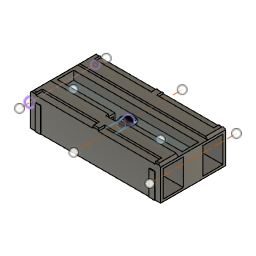
Pièce garage v32 (Autodesk Fusion 360 design; units mm, degrees)
Autodesk Fusion 360 part; units mm, degrees
sketch "Esquisse3" plane through (0, 0, 0) normal (0, 0, 1) x (1, 0, 0)
  line L0 (60, -30) -> (-60, -30)
  line L1 (-60, -30) -> (-60, 30)
  line L2 (-60, 30) -> (60, 30)
  line L3 (60, 30) -> (60, -30)
  line L4 (60, -30) -> (-60, 30) construction
  line L5 (-60, -30) -> (60, 30) construction
  dimension "d3" = 120
  dimension "d4" = 60
  constraint horizontal L0
  constraint perpendicular L0 L1
  constraint parallel L0 L2
  constraint parallel L1 L3
  constraint coincident L4 origin
  constraint coincident L5 origin
  measures "d3" distance of L1.end L2.end
  measures "d4" distance of L0.end L1.end
extrude "Extrusion1" add sketch "Esquisse3" along normal blind 30.7
sketch "Esquisse4" plane through (0, 0, 30.7) normal (0, 0, 1) x (-1, 0, 0)
  line L0 (-60, -30) -> (60, -30)
  line L1 (60, -30) -> (60, 30)
  line L2 (60, 30) -> (-60, 30)
  line L3 (-60, 30) -> (-60, -30)
  line L4 (57.5, 7.5) -> (-57.5, 7.5)
  line L5 (-57.5, 7.5) -> (-57.5, -7.5)
  line L6 (-57.5, -7.5) -> (57.5, -7.5)
  line L7 (57.5, -7.5) -> (57.5, 7.5)
  line L8 (57.5, 7.5) -> (-57.5, -7.5) construction
  line L9 (-57.5, 7.5) -> (57.5, -7.5) construction
  dimension "d7" = 115
  dimension "d8" = 15
  constraint horizontal L4
  constraint perpendicular L4 L5
  constraint parallel L4 L6
  constraint parallel L5 L7
  constraint coincident L8 origin
  constraint coincident L9 origin
  measures "d7" distance of L5.end L6.end
  measures "d8" distance of L4.end L5.end
extrude "Extrusion2" cut sketch "Esquisse4" against normal blind 10 contours L4 L5 L6 L7
sketch "Esquisse5" plane through (0, 0, 20.7) normal (0, 0, 1) x (-1, 0, 0)
  line L0 (57.5, -7.5) -> (57.5, 7.5)
  line L1 (57.5, 7.5) -> (-57.5, 7.5)
  line L2 (-57.5, 7.5) -> (-57.5, -7.5)
  line L3 (-57.5, -7.5) -> (57.5, -7.5)
  circle A0 centre (0, 0) radius 6.15
  circle A1 centre (50.4, 0) radius 3.1
  spline S0 degree 5 poles (60, -40) (60, -36.8) (60, -30.4) (60, -20.8) (60, -8) (60, 8) (60, 20.8) (60, 30.4) (60, 36.8) (60, 40) knots 0 0 0 0 0 0 0.2 0.4 0.6 0.8 1 1 1 1 1 1 construction
  line L4 (60, 30) -> (60, -30) construction
  circle A2 centre (-30, 0) radius 3.1
  spline S1 degree 5 poles (-60, -40) (-60, -36.8) (-60, -30.4) (-60, -20.8) (-60, -8) (-60, 8) (-60, 20.8) (-60, 30.4) (-60, 36.8) (-60, 40) knots 0 0 0 0 0 0 0.2 0.4 0.6 0.8 1 1 1 1 1 1 construction
  line L5 (-60, 31.84) -> (-60, 48.16)
  line L6 (0, -50) -> (0, 50) construction
  line L7 (-4.45, 16) -> (4.45, 16)
  line L8 (4.45, 16) -> (4.45, -3.7)
  line L9 (4.45, -3.7) -> (-4.45, -3.7)
  line L10 (-4.45, -3.7) -> (-4.45, 16)
  line L11 (-4.45, 16) -> (4.45, -3.7) construction
  line L12 (4.45, 16) -> (-4.45, -3.7) construction
  point P0 (0, 6.15)
  dimension "d11" = 12.3
  dimension "d12" = 6.2
  dimension "d13" = 9.6
  dimension "d14" = 6.2
  dimension "d15" = 30
  dimension "d16" = 8.9
  dimension "d17" = 16
  constraint coincident A0.centre origin
  constraint midpoint S1.end L5
  constraint vertical L6
  constraint horizontal L7
  constraint perpendicular L7 L8
  constraint parallel L7 L9
  constraint parallel L8 L10
  constraint coincident L11 P0
  constraint coincident L12 P0
  constraint coincident A0 P0
  constraint coincident L6 P0
  measures "d11" diameter of A0
  measures "d12" diameter of A1
  measures "d13" distance of A1.centre L4
  measures "d14" diameter of A2
  measures "d15" distance of A2.centre L5
  measures "d16" distance of L8.end L9.end
  measures "d17" distance of L7 A0.centre
extrude "Extrusion3" cut sketch "Esquisse5" against normal blind 30.574 contours A1
extrude "Extrusion4" cut sketch "Esquisse5" against normal blind 30.574 contours A0 L8 L9 L10 picked at (-0.0399, -4.5163)
extrude "Extrusion5" cut sketch "Esquisse5" against normal blind 30.574 contours A0 L8 L9 L10 picked at (-0.1506, -0.4222)
extrude "Extrusion6" cut sketch "Esquisse5" against normal blind 30.574 contours L1 A0 L8 L10
extrude "Extrusion7" cut sketch "Esquisse5" against normal blind 30.574 contours L1 L7 L8 L10
extrude "Extrusion8" cut sketch "Esquisse5" along normal blind 22.36 contours L1 L7 L8 L10
extrude "Extrusion9" cut sketch "Esquisse5" against normal blind 30.574 contours A2
sketch "Esquisse6" plane through (0, 0, 30.7) normal (0, 0, 1) x (-1, 0, 0)
  line L0 (-60, -30) -> (60, -30)
  line L1 (60, -30) -> (60, 30)
  line L2 (60, 30) -> (-60, 30)
  line L3 (-60, 30) -> (-60, -30)
  line L4 (-4.45, 7.5) -> (-4.45, 16)
  line L5 (-4.45, 16) -> (4.45, 16)
  line L6 (4.45, 16) -> (4.45, 7.5)
  line L7 (4.45, 7.5) -> (57.5, 7.5)
  line L8 (57.5, 7.5) -> (57.5, -7.5)
  line L9 (57.5, -7.5) -> (-57.5, -7.5)
  line L10 (-57.5, -7.5) -> (-57.5, 7.5)
  line L11 (-57.5, 7.5) -> (-4.45, 7.5)
  line L12 (-60, -13.5) -> (60, -13.5)
  line L13 (60, -13.5) -> (60, 13.5)
  line L14 (60, 13.5) -> (-60, 13.5)
  line L15 (-60, 13.5) -> (-60, -13.5)
  line L16 (-60, -13.5) -> (60, 13.5) construction
  line L17 (60, -13.5) -> (-60, 13.5) construction
  line L18 (0, -50) -> (0, 50) construction
  line L19 (2.5, -50) -> (2.5, 50) construction
  line L20 (-2.5, -50) -> (-2.5, 50) construction
  line L21 (60, -50) -> (60, 50) construction
  line L22 (-60, -50) -> (-60, 50) construction
  line L23 (-60, -50) -> (-60, 50) construction
  line L24 (-55, -50) -> (-55, 50) construction
  line L25 (60, -50) -> (60, 50) construction
  line L26 (55, -50) -> (55, 50) construction
  line L27 (55, -30) -> (2.5, -30)
  line L28 (2.5, -30) -> (2.5, -24)
  line L29 (2.5, -24) -> (55, -24)
  line L30 (55, -24) -> (55, -30)
  line L31 (-2.5, -30) -> (-55, -30)
  line L32 (-55, -30) -> (-55, -24)
  line L33 (-55, -24) -> (-2.5, -24)
  line L34 (-2.5, -24) -> (-2.5, -30)
  line L35 (55, 30) -> (2.5, 30)
  line L36 (2.5, 30) -> (2.5, 24)
  line L37 (2.5, 24) -> (55, 24)
  line L38 (55, 24) -> (55, 30)
  line L39 (-2.5, 30) -> (-55, 30)
  line L40 (-55, 30) -> (-55, 24)
  line L41 (-55, 24) -> (-2.5, 24)
  line L42 (-2.5, 24) -> (-2.5, 30)
  dimension "d32" = 120
  dimension "d33" = 27
  dimension "d34" = 6
  dimension "d35" = 6
  dimension "d36" = 6
  dimension "d37" = 6
  constraint horizontal L12
  constraint perpendicular L12 L13
  constraint parallel L12 L14
  constraint parallel L13 L15
  constraint coincident L16 origin
  constraint coincident L17 origin
  constraint perpendicular L14 L18
  constraint perpendicular L2 L21
  constraint horizontal L27
  constraint vertical L28
  constraint horizontal L29
  constraint vertical L30
  constraint coincident L26 L27.start
  constraint coincident L0 L27.start
  constraint horizontal L31
  constraint vertical L32
  constraint horizontal L33
  constraint vertical L34
  constraint coincident L20 L31.start
  constraint coincident L0 L31.start
  constraint horizontal L35
  constraint vertical L36
  constraint horizontal L37
  constraint vertical L38
  constraint coincident L26 L35.start
  constraint coincident L2 L35.start
  constraint horizontal L39
  constraint vertical L40
  constraint horizontal L41
  constraint vertical L42
  constraint coincident L20 L39.start
  constraint coincident L2 L39.start
  measures "d32" distance of L13.end L14.end
  measures "d33" distance of L12.end L13.end
  measures "d34" distance of L27.start L29.end
  measures "d35" distance of L31.start L33.end
  measures "d36" distance of L35.start L37.end
  measures "d37" distance of L39.start L41.end
extrude "Extrusion10" cut sketch "Esquisse6" against normal blind 2 contours L0 L27 L28 L29 L30
extrude "Extrusion12" cut sketch "Esquisse6" against normal blind 2 contours L0 L31 L32 L33 L34
extrude "Extrusion13" cut sketch "Esquisse6" against normal blind 2 contours L2 L39 L40 L41 L42
extrude "Extrusion14" cut sketch "Esquisse6" against normal blind 2 contours L2 L35 L36 L37 L38
extrude "Extrusion15" cut sketch "Esquisse6" against normal blind 2 contours L1 L3 L4 L6 L7 L8 L9 L10 L11 L12 L13 L14 L15
sketch "Esquisse8" plane through (60, 0, 0) normal (1, 0, 0) x (0, 1, 0)
  line L0 (-13.5, 28.7) -> (-13.5, 30.7)
  line L1 (-13.5, 30.7) -> (-30, 30.7)
  line L2 (-30, 30.7) -> (-30, 0)
  line L3 (-30, 0) -> (30, 0)
  line L4 (30, 0) -> (30, 30.7)
  line L5 (30, 30.7) -> (13.5, 30.7)
  line L6 (13.5, 30.7) -> (13.5, 28.7)
  line L7 (13.5, 28.7) -> (-13.5, 28.7)
  line L8 (-40, 26.5) -> (40, 26.5) construction
  line L9 (-40.0872, 2.1) -> (40, 2.1) construction
  line L10 (27.5, 40.0232) -> (27.5, -9.9768) construction
  line L11 (-27.5, -10) -> (-27.5, 40) construction
  line L12 (9, 40.0232) -> (9, -10) construction
  line L13 (-9, 40) -> (-9, -10) construction
  line L14 (-27.5, 26.5) -> (-9, 26.5)
  line L15 (-9, 26.5) -> (-9, 2.1)
  line L16 (-9, 2.1) -> (-27.5, 2.1)
  line L17 (-27.5, 2.1) -> (-27.5, 26.5)
  line L18 (9, 2.1) -> (27.5, 2.1)
  line L19 (27.5, 2.1) -> (27.5, 26.5)
  line L20 (27.5, 26.5) -> (9, 26.5)
  line L21 (9, 26.5) -> (9, 2.1)
  dimension "d50" = 4.2
  dimension "d51" = 2.1
  dimension "d52" = 2.5
  dimension "d53" = 2.5
  dimension "d54" = 18.5
  dimension "d55" = 18.5
  constraint horizontal L8
  constraint perpendicular L4 L9
  constraint perpendicular L3 L10
  constraint perpendicular L1 L11
  constraint parallel L10 L12
  constraint vertical L13
  constraint horizontal L14
  constraint vertical L15
  constraint horizontal L16
  constraint vertical L17
  constraint coincident L13 L15.end
  constraint coincident L9 L15.end
  constraint coincident L11 L14.start
  constraint coincident L8 L14.start
  constraint horizontal L18
  constraint vertical L19
  constraint horizontal L20
  constraint vertical L21
  constraint coincident L8 L19.end
  constraint coincident L10 L19.end
  constraint coincident L9 L18.start
  constraint coincident L12 L18.start
  measures "d50" distance of L1 L8
  measures "d51" distance of L3 L9
  measures "d52" distance of L4 L10
  measures "d53" distance of L2 L11
  measures "d54" distance of L10.start L12.start
  measures "d55" distance of L11 L13
extrude "Extrusion16" cut sketch "Esquisse8" against normal blind 120 contours L14 L15 L16 L17
extrude "Extrusion17" cut sketch "Esquisse8" against normal blind 120 contours L18 L19 L20 L21
sketch "Esquisse9" plane through (0, -30, 0) normal (0, -1, 0) x (1, 0, 0)
  line L0 (-55, 28.7) -> (-55, 30.7)
  line L1 (-55, 30.7) -> (-60, 30.7)
  line L2 (-60, 30.7) -> (-60, 0)
  line L3 (-60, 0) -> (60, 0)
  line L4 (60, 0) -> (60, 30.7)
  line L5 (60, 30.7) -> (55, 30.7)
  line L6 (55, 30.7) -> (55, 28.7)
  line L7 (55, 28.7) -> (2.5, 28.7)
  line L8 (2.5, 28.7) -> (2.5, 30.7)
  line L9 (2.5, 30.7) -> (-2.5, 30.7)
  line L10 (-2.5, 30.7) -> (-2.5, 28.7)
  line L11 (-2.5, 28.7) -> (-55, 28.7)
  line L12 (-55, 50) -> (-55, -20) construction
  line L13 (-50.2, 50) -> (-50.2, -20) construction
  line L14 (-75, 0) -> (75, 0) construction
  line L15 (-75, 23) -> (75, 23) construction
  line L16 (-50.2, 50) -> (-50.2, -20) construction
  line L17 (-55, 50) -> (-55, -20) construction
  line L18 (55, 50) -> (55, -20) construction
  line L19 (49.8, 50) -> (49.8, -20) construction
  line L20 (-55, 23) -> (-50.2, 23)
  line L21 (-50.2, 23) -> (-50.2, 0)
  line L22 (-50.2, 0) -> (-55, 0)
  line L23 (-55, 0) -> (-55, 23)
  line L24 (55, 0) -> (49.8, 0)
  line L25 (49.8, 0) -> (49.8, 23)
  line L26 (49.8, 23) -> (55, 23)
  line L27 (55, 23) -> (55, 0)
  dimension "d60" = 4.8
  dimension "d61" = 23
  dimension "d62" = 4.8
  constraint perpendicular L11 L12
  constraint perpendicular L11 L13
  constraint parallel L3 L14
  constraint perpendicular L4 L15
  constraint horizontal L20
  constraint vertical L21
  constraint horizontal L22
  constraint vertical L23
  constraint coincident L14 L21.end
  constraint coincident L13 L21.end
  constraint coincident L3 L21.end
  constraint coincident L15 L20.start
  constraint coincident L12 L20.start
  constraint horizontal L24
  constraint vertical L25
  constraint horizontal L26
  constraint vertical L27
  constraint coincident L15 L25.end
  constraint coincident L19 L25.end
  constraint coincident L14 L24.start
  constraint coincident L18 L24.start
  measures "d60" distance of L12 L13
  measures "d61" distance of L14 L15
  measures "d62" distance of L16 L17
extrude "Extrusion18" add sketch "Esquisse9" along normal blind 0.5 contours L3 L24 L25 L26 L27
extrude "Extrusion19" add sketch "Esquisse9" along normal blind 0.5 contours L3 L20 L21 L22 L23
sketch "Esquisse10" plane through (0, 30, 0) normal (0, 1, 0) x (-1, 0, 0)
  line L0 (-2.5, 30.7) -> (-2.5, 28.7)
  line L1 (-2.5, 28.7) -> (-55, 28.7)
  line L2 (-55, 28.7) -> (-55, 30.7)
  line L3 (-55, 30.7) -> (-60, 30.7)
  line L4 (-60, 30.7) -> (-60, 0)
  line L5 (-60, 0) -> (60, 0)
  line L6 (60, 0) -> (60, 30.7)
  line L7 (60, 30.7) -> (55, 30.7)
  line L8 (55, 30.7) -> (55, 28.7)
  line L9 (55, 28.7) -> (2.5, 28.7)
  line L10 (2.5, 28.7) -> (2.5, 30.7)
  line L11 (2.5, 30.7) -> (-2.5, 30.7)
  line L12 (-75, 0) -> (75, 0) construction
  line L13 (-55, 35) -> (-55, -5)
  line L14 (-50, 50) -> (-50, -20) construction
  line L15 (-55, 50) -> (-55, -20) construction
  line L16 (55, 50) -> (55, -20) construction
  line L17 (50, 50) -> (50, -20) construction
  line L18 (-74.8741, 23.108) -> (75, 23.108) construction
  line L19 (-55, 23.108) -> (-50, 23.108)
  line L20 (-50, 23.108) -> (-50, 0)
  line L21 (-50, 0) -> (-55, 0)
  line L22 (-55, 0) -> (-55, 23.108)
  line L23 (50, 23.108) -> (55, 23.108)
  line L24 (55, 23.108) -> (55, 0)
  line L25 (55, 0) -> (50, 0)
  line L26 (50, 0) -> (50, 23.108)
  constraint perpendicular L6 L12
  constraint perpendicular L3 L13
  constraint vertical L14
  constraint vertical L15
  constraint vertical L17
  constraint vertical L16
  constraint perpendicular L16 L18
  constraint horizontal L19
  constraint vertical L20
  constraint horizontal L21
  constraint vertical L22
  constraint coincident L12 L20.end
  constraint coincident L14 L20.end
  constraint coincident L5 L20.end
  constraint coincident L13 L19.start
  constraint coincident L18 L19.start
  constraint horizontal L23
  constraint vertical L24
  constraint horizontal L25
  constraint vertical L26
  constraint coincident L12 L24.end
  constraint coincident L16 L24.end
  constraint coincident L17 L23.start
  constraint coincident L18 L23.start
extrude "Extrusion20" add sketch "Esquisse10" along normal blind 0.5 contours L5 L23 L24 L25 L26
extrude "Extrusion21" add sketch "Esquisse10" along normal blind 0.5 contours L5 L13 L19 L20 L21 L22
sketch "Esquisse11" plane through (0, 0, 0) normal (0, 0, -1) x (1, 0, 0)
  circle A0 centre (30, 0) radius 3.1
  line L0 (4.45, 16) -> (4.45, 4.245)
  arc A1 (-4.45, 4.245) -> (4.45, 4.245) centre (0, 0) ccw
  line L1 (-4.45, 4.245) -> (-4.45, 16)
  line L2 (-4.45, 16) -> (4.45, 16)
  line L3 (-60, -30) -> (-55, -30)
  line L4 (-55, -30) -> (-55, -30.5)
  line L5 (-55, -30.5) -> (-50, -30.5)
  line L6 (-50, -30.5) -> (-50, -30)
  line L7 (-50, -30) -> (50, -30)
  line L8 (50, -30) -> (50, -30.5)
  line L9 (50, -30.5) -> (55, -30.5)
  line L10 (55, -30.5) -> (55, -30)
  line L11 (55, -30) -> (60, -30)
  line L12 (60, -30) -> (60, 30)
  line L13 (60, 30) -> (55, 30)
  line L14 (55, 30) -> (55, 30.5)
  line L15 (55, 30.5) -> (49.8, 30.5)
  line L16 (49.8, 30.5) -> (49.8, 30)
  line L17 (49.8, 30) -> (-50.2, 30)
  line L18 (-50.2, 30) -> (-50.2, 30.5)
  line L19 (-50.2, 30.5) -> (-55, 30.5)
  line L20 (-55, 30.5) -> (-55, 30)
  line L21 (-55, 30) -> (-60, 30)
  line L22 (-60, 30) -> (-60, -30)
  circle A2 centre (-50.4, 0) radius 3.1
  line L23 (-75, 28) -> (70, 28) construction
  line L24 (-75, -28) -> (70, -28) construction
  line L25 (75, -30) -> (-75, -30)
  line L26 (-55, 40) -> (-55, -40) construction
  line L27 (55, 40) -> (55, -40) construction
  line L28 (-75, 23) -> (70, 23) construction
  line L29 (-75, 23) -> (70, 23) construction
  line L30 (-75, -23) -> (70, -23) construction
  line L31 (-45, 40) -> (-45, -45) construction
  line L32 (45, 40) -> (45, -45) construction
  line L33 (-55, 28) -> (-45, 28)
  line L34 (-45, 28) -> (-45, 23)
  line L35 (-45, 23) -> (-55, 23)
  line L36 (-55, 23) -> (-55, 28)
  line L37 (-55, -23) -> (-45, -23)
  line L38 (-45, -23) -> (-45, -28)
  line L39 (-45, -28) -> (-55, -28)
  line L40 (-55, -28) -> (-55, -23)
  line L41 (45, -23) -> (55, -23)
  line L42 (55, -23) -> (55, -28)
  line L43 (55, -28) -> (45, -28)
  line L44 (45, -28) -> (45, -23)
  line L45 (45, 28) -> (55, 28)
  line L46 (55, 28) -> (55, 23)
  line L47 (55, 23) -> (45, 23)
  line L48 (45, 23) -> (45, 28)
  dimension "d73" = 2
  dimension "d74" = 2
  dimension "d75" = 5
  dimension "d76" = 5
  dimension "d78" = 5
  dimension "d79" = 5
  dimension "d80" = 10
  dimension "d81" = 10
  constraint perpendicular L12 L23
  constraint perpendicular L25 L26
  constraint perpendicular L25 L27
  constraint perpendicular L12 L28
  constraint perpendicular L25 L31
  constraint horizontal L33
  constraint vertical L34
  constraint horizontal L35
  constraint vertical L36
  constraint coincident L28 L34.end
  constraint coincident L31 L34.end
  constraint coincident L23 L33.start
  constraint coincident L26 L33.start
  constraint horizontal L37
  constraint vertical L38
  constraint horizontal L39
  constraint vertical L40
  constraint coincident L31 L38.end
  constraint coincident L24 L38.end
  constraint coincident L30 L37.start
  constraint coincident L26 L37.start
  constraint horizontal L41
  constraint vertical L42
  constraint horizontal L43
  constraint vertical L44
  constraint coincident L24 L42.end
  constraint coincident L27 L42.end
  constraint coincident L30 L41.start
  constraint coincident L32 L41.start
  constraint horizontal L45
  constraint vertical L46
  constraint horizontal L47
  constraint vertical L48
  constraint coincident L28 L46.end
  constraint coincident L27 L46.end
  constraint coincident L32 L45.start
  constraint coincident L23 L45.start
  measures "d73" distance of L21 L23
  measures "d74" distance of L24 L25
  measures "d75" distance of L22 L26
  measures "d76" distance of L12 L27
  measures "d78" distance of L23 L28
  measures "d79" distance of L24 L30
  measures "d80" distance of L26 L31
  measures "d81" distance of L27 L32
extrude "Extrusion23" add sketch "Esquisse11" along normal blind 0.5 contours L33 L34 L35 L36 | L37 L38 L39 L40 | L41 L42 L43 L44 | L45 L46 L47 L48
sketch "Esquisse12" plane through (0, 0, 0) normal (0, 0, -1) x (1, 0, 0)
  line L0 (45, 23) -> (45, 28)
  line L1 (45, 28) -> (55, 28)
  line L2 (55, 28) -> (55, 23)
  line L3 (55, 23) -> (45, 23)
  line L4 (-55, 23) -> (-55, 28)
  line L5 (-55, 28) -> (-45, 28)
  line L6 (-45, 28) -> (-45, 23)
  line L7 (-45, 23) -> (-55, 23)
  line L8 (45, -28) -> (45, -23)
  line L9 (45, -23) -> (55, -23)
  line L10 (55, -23) -> (55, -28)
  line L11 (55, -28) -> (45, -28)
  line L12 (-55, -28) -> (-55, -23)
  line L13 (-55, -23) -> (-45, -23)
  line L14 (-45, -23) -> (-45, -28)
  line L15 (-45, -28) -> (-55, -28)
  circle A0 centre (30, 0) radius 3.1
  line L16 (4.45, 16) -> (4.45, 4.245)
  arc A1 (-4.45, 4.245) -> (4.45, 4.245) centre (0, 0) ccw
  line L17 (-4.45, 4.245) -> (-4.45, 16)
  line L18 (-4.45, 16) -> (4.45, 16)
  line L19 (-60, -30) -> (-55, -30)
  line L20 (-55, -30) -> (-55, -30.5)
  line L21 (-55, -30.5) -> (-50, -30.5)
  line L22 (-50, -30.5) -> (-50, -30)
  line L23 (-50, -30) -> (50, -30)
  line L24 (50, -30) -> (50, -30.5)
  line L25 (50, -30.5) -> (55, -30.5)
  line L26 (55, -30.5) -> (55, -30)
  line L27 (55, -30) -> (60, -30)
  line L28 (60, -30) -> (60, 30)
  line L29 (60, 30) -> (55, 30)
  line L30 (55, 30) -> (55, 30.5)
  line L31 (55, 30.5) -> (49.8, 30.5)
  line L32 (49.8, 30.5) -> (49.8, 30)
  line L33 (49.8, 30) -> (-50.2, 30)
  line L34 (-50.2, 30) -> (-50.2, 30.5)
  line L35 (-50.2, 30.5) -> (-55, 30.5)
  line L36 (-55, 30.5) -> (-55, 30)
  line L37 (-55, 30) -> (-60, 30)
  line L38 (-60, 30) -> (-60, -30)
  circle A2 centre (-50.4, 0) radius 3.1
  line L39 (-58, 35) -> (-58, -35) construction
  line L40 (-43, 35) -> (-43, -35) construction
  line L41 (-70, -7) -> (70, -7) construction
  line L42 (-70, 7) -> (70, 7) construction
  line L43 (23, 35) -> (23, -35) construction
  line L44 (38, 35) -> (38, -35) construction
  line L45 (-58, 7) -> (-43, 7)
  line L46 (-43, 7) -> (-43, -7)
  line L47 (-43, -7) -> (-58, -7)
  line L48 (-58, -7) -> (-58, 7)
  line L49 (23, 7) -> (38, 7)
  line L50 (38, 7) -> (38, -7)
  line L51 (38, -7) -> (23, -7)
  line L52 (23, -7) -> (23, 7)
  line L53 (60, -40) -> (60, 40)
  point P0 (30, 0)
  dimension "d84" = 2
  dimension "d85" = 15
  dimension "d86" = 23
  dimension "d87" = 23
  dimension "d90" = 22
  dimension "d91" = 30
  dimension "d92" = 30
  constraint parallel L38 L39
  constraint perpendicular L21 L40
  constraint perpendicular L28 L41
  constraint horizontal L45
  constraint vertical L46
  constraint horizontal L47
  constraint vertical L48
  constraint coincident L40 L46.end
  constraint coincident L41 L46.end
  constraint coincident L42 L45.start
  constraint coincident L39 L45.start
  constraint horizontal L49
  constraint vertical L50
  constraint horizontal L51
  constraint vertical L52
  constraint coincident L41 L50.end
  constraint coincident L44 L50.end
  constraint coincident L42 L49.start
  constraint coincident L43 L49.start
  measures "d84" distance of L38 L39
  measures "d85" distance of L39 L40
  measures "d86" distance of L23 L41
  measures "d87" distance of L33 L42
  measures "d90" distance of L28 L44
  measures "d91" distance of P0 L53
  measures "d92" distance of P0 L53
extrude "Extrusion24" cut sketch "Esquisse12" against normal blind 6 contours L45 L46 L47 L48 | L49 L50 L51 L52
sketch "Esquisse13" plane through (0, 0, 6) normal (0, 0, -1) x (1, 0, 0)
  circle A0 centre (30, 0) radius 3.1
  line L0 (23, -7) -> (38, -7)
  line L1 (38, -7) -> (38, 7)
  line L2 (38, 7) -> (23, 7)
  line L3 (23, 7) -> (23, -7)
  line L4 (35.4725, -1.8397) -> (34.3295, 3.8195)
  line L5 (34.3295, 3.8195) -> (28.857, 5.6592)
  line L6 (28.857, 5.6592) -> (24.5275, 1.8397)
  line L7 (24.5275, 1.8397) -> (25.6705, -3.8195)
  line L8 (25.6705, -3.8195) -> (31.143, -5.6592)
  line L9 (31.143, -5.6592) -> (35.4725, -1.8397)
  point P0 (30, 0)
  dimension "d95" = 5
  constraint coincident P0 A0.centre
  measures "d95" distance of P0 L9
extrude "Extrusion25" cut sketch "Esquisse13" against normal blind 5 contours L4 L5 L6 L7 L8 L9
sketch "Esquisse14" plane through (0, 0, 6) normal (0, 0, -1) x (1, 0, 0)
  circle A0 centre (-50.4, 0) radius 3.1
  line L0 (-58, -7) -> (-43, -7)
  line L1 (-43, -7) -> (-43, 7)
  line L2 (-43, 7) -> (-58, 7)
  line L3 (-58, 7) -> (-58, -7)
  line L4 (-44.7702, -1.2801) -> (-46.4765, 4.2355)
  line L5 (-46.4765, 4.2355) -> (-52.1063, 5.5156)
  line L6 (-52.1063, 5.5156) -> (-56.0298, 1.2801)
  line L7 (-56.0298, 1.2801) -> (-54.3235, -4.2355)
  line L8 (-54.3235, -4.2355) -> (-48.6937, -5.5156)
  line L9 (-48.6937, -5.5156) -> (-44.7702, -1.2801)
  point P0 (-50.4, 0)
  dimension "d98" = 5
  constraint coincident P0 A0.centre
  measures "d98" distance of P0 L9
extrude "Extrusion26" cut sketch "Esquisse14" against normal blind 5 contours L4 L5 L6 L7 L8 L9
chamfer "Chanfrein1" distance 2 angle 45 1 edges at (60, -21.75, 30.7)
chamfer "Chanfrein2" distance 2 angle 45 1 edges at (60, 21.75, 30.7)
chamfer "Chanfrein3" distance 2 angle 45 1 edges at (-60, 21.75, 30.7)
chamfer "Chanfrein4" distance 2 angle 45 1 edges at (-60, -21.75, 30.7)
fillet "Congé1" radius 1.5 3 edges at (56.5, 30, 30.7) (0, 30, 30.7) (-56.5, 30, 30.7)
fillet "Congé2" radius 1 tangency weight 1.5 3 edges at (-56.5, -30, 30.7) (0, -30, 30.7) (56.5, -30, 30.7)
extrude "Extrusion22" [suppressed]
extrude "Extrusion11" [suppressed]
